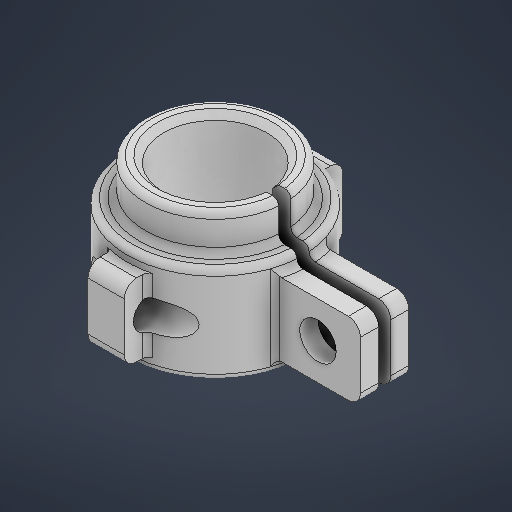
# Autodesk Inventor part: Sup_motor_coreless
Saved by Autodesk Inventor 2026.1 (Build 301233020, 233B)
## iProperties
Created: 2026-03-24
Part Number: Sup_motor_coreless
Material: Genérico
Document SubType Name: Modeling
Designer: celio
Density: 1 g/cm^3
Appearance: Padrão
Author: celio
Autodesk Inventor part; units mm, degrees
ref_plane "YZ Plane" through (0, 0, 0) normal (1, 0, 0) x (0, 1, 0)
ref_plane "XZ Plane" through (0, 0, 0) normal (0, 1, 0) x (-1, 0, 0)
sketch "Esboço2" plane through (0, 0, 0) normal (0, 1, 0) x (-1, 0, 0)
  circle A0 centre (0, 0) radius 4.25
  circle A1 centre (0, 0) radius 7.25
  dimension "d4" = 8.5
  dimension "d5" = 3
  constraints: 2 centre point, 1 coincident
  measures "d4" diameter of A0
  measures "d5" radial gap between concentric circles of A0 A1
extrude "Extrusão1" add sketch "Esboço2" along normal blind 8
sketch "Esboço3" plane through (0, 8, 0) normal (0, 1, 0) x (1, 0, 0)
  circle A0 centre (0, 0) radius 4.25
  circle A1 centre (0, 0) radius 5.75
  dimension "d8" = 8.5
  dimension "d9" = 1.5
  constraints: 2 centre point, 1 coincident
  measures "d8" diameter of A0
  measures "d9" radial gap between concentric circles of A0 A1
extrude "Extrusão2" add sketch "Esboço3" along normal blind 3
sketch "Esboço4" plane through (0, 11, 0) normal (0, 1, 0) x (1, 0, 0)
  line L0 (2.75, -0.5) -> (8.75, -0.5)
  line L1 (8.75, -0.5) -> (8.75, 0.5)
  line L2 (8.75, 0.5) -> (2.75, 0.5)
  line L3 (2.75, 0.5) -> (2.75, -0.5)
  circle A0 centre (0, 0) radius 5.75 projected
  line L4 (2.75, -0.5) -> (8.75, 0.5) construction
  line L5 (8.75, -0.5) -> (2.75, 0.5) construction
  point P0 (5.75, 0)
  dimension "d12" = 6
  dimension "d13" = 1
  constraints: 12 end point, 2 midpoint, 2 parallel, 1 horizontal, 1 horizontal alignment, 1 perpendicular, 1 other
  measures "d12" distance of L2.end L1.end
  measures "d13" distance of L1.end L0.end
extrude "Extrusão3" cut sketch "Esboço4" against normal through all contours L3 L2 A0 L0 | A0 L2 L1 L0 picked at (3.75, 0)
ref_plane "Plano de trabalho1" through (0, 4, 0) normal (0, -1, 0) x (1, 0, 0)
sketch "Esboço5" plane through (0, 4, 0) normal (0, -1, 0) x (1, 0, 0)
  line L0 (4.2205, 0.5) -> (7.2327, 0.5) projected
  line L1 (5.7266, 0.5) -> (14.7266, 0.5)
  line L2 (14.7266, 0.5) -> (14.7266, -0.5)
  line L3 (14.7266, -0.5) -> (5.7266, -0.5)
  line L4 (5.7266, -0.5) -> (5.7266, 0.5)
  line L5 (14.7266, 2) -> (4.2266, 2)
  line L6 (4.2266, 2) -> (4.2266, -2)
  line L7 (4.2266, -2) -> (14.7266, -2)
  line L8 (7.2327, -0.5) -> (4.2205, -0.5) projected
  line L9 (5.7266, -0.5) -> (4.2205, -0.5)
  line L10 (5.7266, -0.5) -> (4.2205, -0.5)
  line L11 (14.7266, -2) -> (14.7266, 2)
  point P0 (0, 0)
  point P1 (11.7266, -2)
  point P2 (11.7266, 2)
  point P3 (4.2266, 0.5)
  point P4 (4.2266, -0.5)
  dimension "d16" = 9
  dimension "d17" = 1
  dimension "d18" = 1.5
  constraints: 20 end point, 4 point on line, 3 parallel, 1 horizontal, 1 midpoint, 1 perpendicular, 1 vertical
  measures "d16" distance of L2.end L3.end
  measures "d17" distance of L1.end L2.end
  measures "d18" distance between parallel lines of L1 L5
extrude "Extrusão4" add sketch "Esboço5" along normal mid plane 6 contours L0 L6 L5 L11 L1 | L3 L11 L7 L6 L8
sketch "Esboço7" plane through (6.9687, 1, 2) normal (0, 0, 1) x (1, 0, 0)
  line L0 (0, 6) -> (0, 0) projected
  circle A0 centre (3.5, 3) radius 1.5
  line L1 (3.5, 3) -> (7, 3)
  line L2 (7, 3) -> (7, 6)
  line L3 (0, 0) -> (7.7579, 0) projected
  line L4 (7, 6) -> (7.7579, 6)
  line L5 (7.7579, 6) -> (7.7579, 0)
  line L6 (7.7579, 0) -> (7, 0)
  line L7 (7, 0) -> (7, 6)
  point P0 (-6.9687, -1)
  point P1 (7, 3)
  point P2 (7, 0)
  dimension "d27" = 3
  dimension "d30" = 3.5
  constraints: 12 end point, 2 horizontal, 2 parallel, 2 perpendicular, 1 centre point
  measures "d27" diameter of A0
  measures "d30" distance of L1.start L1.end
extrude "Extrusão7" cut sketch "Esboço7" against normal through all
fillet "Arredondamento2" radius 1 4 edges at (13.9687, 7, -1.25) (13.9687, 7, 1.25) (13.9687, 1, 1.25) (13.9687, 1, -1.25)
sketch "Esboço8" plane through (0, 0, 0) normal (1, 0, 0) x (0, 1, 0)
  line L0 (0, 0) -> (8, 0)
  line L1 (8, 5.75) -> (8, -5.75) projected
  line L2 (7, 7) -> (1, 7)
  line L3 (1, 7) -> (1, -7)
  line L4 (1, -7) -> (7, -7)
  line L5 (7, -7) -> (7, 7)
  line L6 (7, 7) -> (1, -7) construction
  line L7 (1, 7) -> (7, -7) construction
  circle A0 centre (4, -7) radius 1.25
  circle A1 centre (4, 7) radius 1.25
  point P0 (8, 0.5)
  point P1 (8, -0.5)
  point P2 (4, 0)
  dimension "d34" = 6
  dimension "d35" = 14
  dimension "d40" = 2.5
  dimension "d41" = 2.5
  constraints: 14 end point, 6 midpoint, 2 centre point, 2 parallel, 1 horizontal, 1 perpendicular
  measures "d34" distance of L4.end L3.end
  measures "d35" distance of L3.end L2.end
  measures "d40" diameter of A0
  measures "d41" diameter of A1
sketch "Esboço9" plane through (0, 0, 0) normal (0, 0, 1) x (1, 0, 0)
  line L0 (-1.5, 1) -> (1.5, 1)
  line L1 (1.5, 1) -> (1.5, 7)
  line L2 (1.5, 7) -> (-1.5, 7)
  line L3 (-1.5, 7) -> (-1.5, 1)
  line L4 (-1.5, 1) -> (1.5, 7) construction
  line L5 (1.5, 1) -> (-1.5, 7) construction
  point P0 (0, 0)
  point P1 (0, 4)
  dimension "d36" = 3
  dimension "d37" = 6
  constraints: 12 end point, 2 midpoint, 2 parallel, 1 horizontal, 1 perpendicular
  measures "d36" distance of L2.end L1.end
  measures "d37" distance of L1.end L0.end
extrude "Extrusão8" add sketch "Esboço9" along normal mid plane 18
extrude "Extrusão9" cut sketch "Esboço8" along normal through all both and the other way through all contours A1 L2 | L2 A1 | A0 L4 | L4 A0
fillet "Arredondamento3" radius 1 4 edges at (0, 7, -9) (0, 1, -9) (0, 7, 9) (0, 1, 9)
extrude "Extrusão10" cut sketch "Esboço2" along normal through all both and the other way through all contours A0
chamfer "Chanfro1" distance 0.5 angle 45 4 edges at (-0.2504, 11, -4.2426) (-0.2504, 11, 4.2426) (-0.2504, 0, 4.2426) (-0.2504, 0, -4.2426)
fillet "Arredondamento4" radius 0.5 15 edges at (-5.75, 8, 0) (1.5, 6.1233, 7.0931) (1.5, 1.8767, 7.0931) (-1.5, 6.1233, 7.0931) (-1.5, 1.8767, 7.0931) (6.9687, 4, 2) (7.1402, 7, 1.257) (7.1402, 1, 1.257) (7.1402, 1, -1.257) (6.9687, 4, -2) (7.1402, 7, -1.257) (1.5, 6.1233, -7.0931) (1.5, 1.8767, -7.0931) (-1.5, 6.1233, -7.0931) (-1.5, 1.8767, -7.0931)
fillet "Arredondamento5" radius 0.5 1 edges at (-7.25, 8, 0)
fillet "Arredondamento6" radius 0.5 1 edges at (-5.75, 11, 0)
fillet "Arredondamento7" radius 0.5 1 edges at (-7.25, 0, 0)
